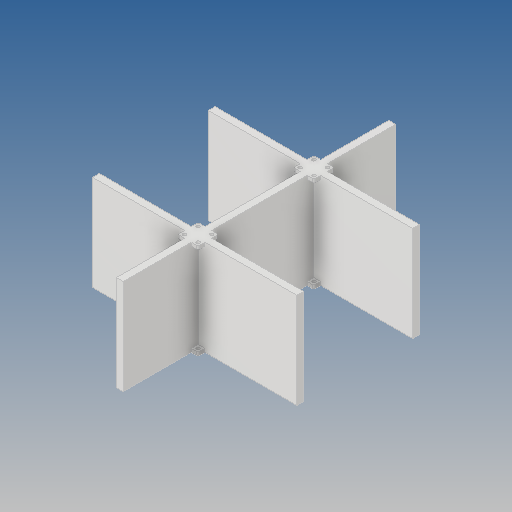
# Autodesk Inventor part: крепление-стенки
Saved by Autodesk Inventor 2020 (Build 240168000, 168)
## iProperties
Created: 2019-10-05
Part Number: крепление-стенки
Material: Пластик АБС
Document SubType Name: Modeling
Designer: Iliga
Density: 1.06 g/cm^3
Appearance: Гладкий — белый
Author: Iliga
Autodesk Inventor part; units mm, degrees
ref_plane "YZ Plane" through (0, 0, 0) normal (1, 0, 0) x (0, 1, 0)
ref_plane "XY Plane" through (0, 0, 0) normal (0, 0, 1) x (1, 0, 0)
sketch "Эскиз1" plane through (0, 0, 0) normal (0, 1, 0) x (-1, 0, 0)
  line L0 (-2, 80) -> (2, 80)
  line L1 (2, 80) -> (2, -80)
  line L2 (2, -80) -> (-2, -80)
  line L3 (-2, -80) -> (-2, 80)
  line L4 (60, 32) -> (-60, 32)
  line L5 (-60, 32) -> (-60, 36)
  line L6 (-60, 36) -> (60, 36)
  line L7 (60, 36) -> (60, 32)
  line L8 (60, -32) -> (-60, -32)
  line L9 (-60, -32) -> (-60, -36)
  line L10 (-60, -36) -> (60, -36)
  line L11 (60, -36) -> (60, -32)
  line L12 (60, 32) -> (60, -32) construction
  line L13 (2, -80) -> (2, -80)
  line L14 (2, -80) -> (-2, -80)
  point P0 (0, 0)
  point P1 (0, -32)
  point P2 (60, 0)
  point P3 (0, -80)
  point P4 (2, 0)
  dimension "d1" = 120
  dimension "d3" = 4
  dimension "d4" = 4
  dimension "d5" = 4
  dimension "d26" = 32
  dimension "d27" = 32
  dimension "d28" = 80
  dimension "d29" = 80
  dimension "d32" = 44
  constraints: 30 end point, 5 parallel, 5 perpendicular, 4 midpoint, 3 horizontal, 3 point on line, 2 vertical alignment, 1 horizontal alignment
  measures "d1" distance between parallel lines of L5 L7
  measures "d3" distance between parallel lines of L6 L4
  measures "d4" distance between parallel lines of L1 L3
  measures "d5" distance between parallel lines of L10 L8
  measures "d26" distance from line of point (0, 0) L8
  measures "d27" distance from line of point (0, 0) L4
  measures "d28" distance from line of L0 point (0, 0)
  measures "d29" distance of point (0, -80) point (0, 0)
  measures "d32" distance from line of L0.start L6
extrude "Выдавливание1" add sketch "Эскиз1" along normal blind 56
ref_plane "РабПлоскость1" through (0, 28, 0) normal (0, 1, 0) x (-1, 0, 0)
sketch "Эскиз2" plane through (0, 0, 0) normal (0, 1, 0) x (-1, 0, 0)
  line L0 (-2, 36) -> (-2, 80) construction
  line L1 (-2, 80) -> (2, 80) construction
  line L2 (2, 80) -> (2, 36) construction
  line L3 (2, 36) -> (60, 36) construction
  line L4 (60, 36) -> (60, 32) construction
  line L5 (60, 32) -> (2, 32) construction
  line L6 (2, 32) -> (2, -32) construction
  line L7 (60, -32) -> (2, -32) construction
  line L8 (60, -36) -> (60, -32) construction
  line L9 (2, -36) -> (60, -36) construction
  line L10 (2, -36) -> (2, -80) construction
  line L11 (2, -80) -> (-2, -80) construction
  line L12 (-2, -80) -> (-2, -36) construction
  line L13 (-60, -36) -> (-2, -36) construction
  line L14 (-60, -32) -> (-60, -36) construction
  line L15 (-2, -32) -> (-60, -32) construction
  line L16 (-2, -32) -> (-2, 32) construction
  line L17 (-2, 32) -> (-60, 32) construction
  line L18 (-60, 32) -> (-60, 36) construction
  line L19 (-60, 36) -> (-2, 36) construction
  line L20 (-2, 32) -> (-6, 32)
  line L21 (-6, 32) -> (-6, 29)
  line L22 (-5, 28) -> (-2, 28)
  line L23 (-2, 28) -> (-2, 32)
  circle A0 centre (-4, 30) radius 1
  arc A1 (-6, 29) -> (-5, 28) centre (-5, 29) ccw
  line L24 (-2, -36) -> (-6, -36)
  line L25 (-6, -36) -> (-6, -39)
  line L26 (-5, -40) -> (-2, -40)
  line L27 (-2, -40) -> (-2, -36)
  circle A2 centre (-4, -38) radius 1
  arc A3 (-6, -39) -> (-5, -40) centre (-5, -39) ccw
  line L28 (-60, 34) -> (60, 34) construction
  line L29 (-60, -34) -> (60, -34) construction
  line L30 (0, 80) -> (0, -80) construction
  line L31 (-2, 36) -> (-6, 36)
  line L32 (-6, 36) -> (-6, 39)
  line L33 (-5, 40) -> (-2, 40)
  line L34 (-2, 40) -> (-2, 36)
  circle A4 centre (-4, 38) radius 1
  arc A5 (-5, 40) -> (-6, 39) centre (-5, 39) ccw
  line L35 (2, 32) -> (6, 32)
  line L36 (6, 32) -> (6, 29)
  line L37 (5, 28) -> (2, 28)
  line L38 (2, 28) -> (2, 32)
  circle A6 centre (4, 30) radius 1
  arc A7 (5, 28) -> (6, 29) centre (5, 29) ccw
  arc A8 (6, 39) -> (5, 40) centre (5, 39) ccw
  line L39 (5, 40) -> (2, 40)
  line L40 (2, 40) -> (2, 36)
  line L41 (6, 36) -> (6, 39)
  line L42 (2, 36) -> (6, 36)
  circle A9 centre (4, 38) radius 1
  line L43 (-2, -28) -> (-2, -32)
  line L44 (-2, -32) -> (-6, -32)
  circle A10 centre (-4, -30) radius 1
  line L45 (-6, -32) -> (-6, -29)
  arc A11 (-5, -28) -> (-6, -29) centre (-5, -29) ccw
  line L46 (-5, -28) -> (-2, -28)
  line L47 (2, -40) -> (2, -36)
  line L48 (2, -36) -> (6, -36)
  circle A12 centre (4, -38) radius 1
  line L49 (6, -36) -> (6, -39)
  arc A13 (5, -40) -> (6, -39) centre (5, -39) ccw
  line L50 (5, -40) -> (2, -40)
  line L51 (2, -28) -> (2, -32)
  line L52 (2, -32) -> (6, -32)
  line L53 (6, -32) -> (6, -29)
  line L54 (5, -28) -> (2, -28)
  arc A14 (6, -29) -> (5, -28) centre (5, -29) ccw
  circle A15 centre (4, -30) radius 1
  point P0 (0, 0)
  point P1 (-6, 28)
  point P2 (-6, -40)
  point P3 (-6, 40)
  point P4 (6, 28)
  point P5 (6, 40)
  point P6 (-6, -28)
  point P7 (2, -32)
  point P8 (6, -40)
  point P9 (6, -28)
  dimension "d11" = 4
  dimension "d12" = 4
  dimension "d13" = 2
  dimension "d15" = 1
  dimension "d16" = 2
  dimension "d17" = 2
  dimension "d18" = 4
  dimension "d19" = 4
  dimension "d20" = 2
  dimension "d21" = 1
  dimension "d22" = 2
  dimension "d23" = 2
  constraints: 70 end point, 49 symmetric about line, 18 point on line, 16 centre point, 16 point on circle, 6 midpoint, 4 parallel, 4 tangent, 2 horizontal, 2 perpendicular, 12 other
  measures "d11" distance of L22.end point (-6, 28)
  measures "d12" distance of point (-6, 28) L20.end
  measures "d13" diameter of A0
  measures "d15" radius of A1
  measures "d16" distance from line of L20 A0.centre
  measures "d17" distance from line of L23 A0.centre
  measures "d18" distance of L27.start point (-6, -40)
  measures "d19" distance of point (-6, -40) L24.end
  measures "d20" diameter of A2
  measures "d21" radius of A3
  measures "d22" distance from line of L24 A2.centre
  measures "d23" distance from line of L27 A2.centre
extrude "Выдавливание2" add sketch "Эскиз2" along normal blind 2
mirror "Зеркальное отражение1" about plane through (0, 28, 0) normal (0, 1, 0) of "Выдавливание2"
extrude "Выдавливание3" add sketch "Эскиз1" along normal up to surface (56 mm away) contours L0 L1 L6 L3 | L6 L1 L4 L3 | L4 L1 L8 L3 | L8 L1 L10 L3 | L10 L1 L2 L3
